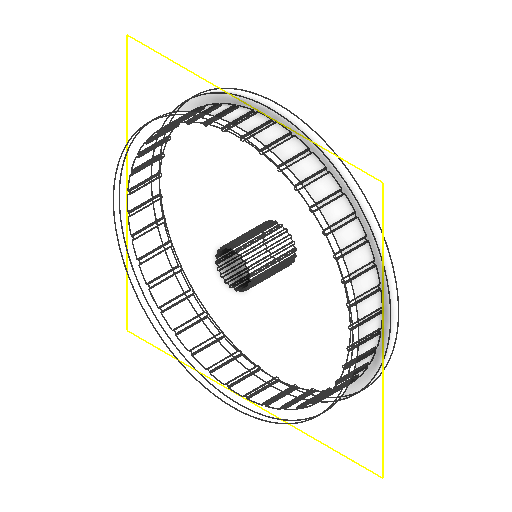
# Autodesk Inventor part: Diff Large Pulley
Saved by Autodesk Inventor 2025.2 (Build 292293000, 293)
## iProperties
Created: 2025-02-20
Part Number: Diff Large Pulley
Material: Generic
Document SubType Name: Modeling
Designer: Jakeg
Density: 1 g/cm^3
Appearance: Default
Author: Jakeg
Autodesk Inventor part; units mm, degrees
ref_plane "YZ Plane" through (0, 0, 0) normal (1, 0, 0) x (0, 1, 0)
ref_plane "XZ Plane" through (0, 0, 0) normal (0, 1, 0) x (-1, 0, 0)
ref_plane "XY Plane" through (0, 0, 0) normal (0, 0, 1) x (1, 0, 0)
sketch "Sketch1" plane through (0, 0, 0) normal (0, 0, 1) x (1, 0, 0)
  circle A0 centre (0, 0) radius 41.14
  dimension "d0" = 82.28
  constraints: 1 centre point, 1 coincident
  measures "d0" diameter of A0
extrude "Extrusion1" add sketch "Sketch1" along normal blind 15.7
ref_plane "Work Plane1" through (0, 0, 8.2) normal (0, 0, 1) x (1, 0, 0)
sketch "Sketch2" plane through (0, 0, 8.2) normal (0, 0, 1) x (1, 0, 0)
  circle A0 centre (0, 0) radius 38.3
  circle A1 centre (0, 0) radius 41.14
  dimension "d4" = 76.6
  constraints: 2 centre point, 2 coincident
  measures "d4" diameter of A0
extrude "Extrusion2" cut sketch "Sketch2" along normal mid plane 11
sketch "Sketch3" plane through (0, 0, 15.7) normal (0, 0, 1) x (1, 0, 0)
  circle A0 centre (0, 0) radius 6
  circle A1 centre (0, 20.32) radius 3.175
  circle A2 centre (0, -20.32) radius 3.175
  dimension "d7" = 12
  dimension "d13" = 6.35
  dimension "d14" = 20.32
  dimension "d15" = 6.35
  dimension "d16" = 20.32
  constraints: 3 centre point, 1 coincident
  measures "d7" diameter of A0
  measures "d13" diameter of A1
  measures "d14" distance of point (0, 0) A1.centre
  measures "d15" diameter of A2
  measures "d16" distance of point (0, 0) A2.centre
extrude "Extrusion3" cut sketch "Sketch3" against normal through all contours A0
sketch "Sketch5" plane through (0, 0, 15.7) normal (0, 0, 1) x (1, 0, 0)
  circle A0 centre (0, 0) radius 6 projected
  arc A1 (-1.2778, -5.5469) -> (-2.2267, -5.2386) centre (-1.8274, -5.6241) ccw
  arc A2 (-1.2783, -5.8289) -> (-1.2778, -5.5469) centre (-2.2681, -5.6859) ccw
  arc A3 (-1.2783, -5.8289) -> (-1.1583, -5.9977) centre (-1.1299, -5.8504) ccw
  arc A4 (-1.1583, -5.9977) -> (-0.7518, -6.0621) centre (0, 0) ccw
  arc A5 (-0.7518, -6.0621) -> (-0.5855, -5.9387) centre (-0.7333, -5.9132) ccw
  arc A6 (-0.4989, -5.6703) -> (-0.5855, -5.9387) centre (0.4, -6.1085) ccw
  arc A7 (0.4989, -5.6703) -> (-0.4989, -5.6703) centre (0, -5.9135) ccw
  arc A8 (0.5855, -5.9387) -> (0.4989, -5.6703) centre (-0.4, -6.1085) ccw
  arc A9 (0.5855, -5.9387) -> (0.7518, -6.0621) centre (0.7333, -5.9132) ccw
  arc A10 (0.7518, -6.0621) -> (1.1583, -5.9977) centre (0, 0) ccw
  arc A11 (1.1583, -5.9977) -> (1.2783, -5.8289) centre (1.1299, -5.8504) ccw
  arc A12 (1.2778, -5.5469) -> (1.2783, -5.8289) centre (2.2681, -5.6859) ccw
  arc A13 (2.2267, -5.2386) -> (1.2778, -5.5469) centre (1.8274, -5.6241) ccw
  arc A14 (2.392, -5.4671) -> (2.2267, -5.2386) centre (1.5072, -5.9331) ccw
  arc A15 (2.392, -5.4671) -> (2.5882, -5.5331) centre (2.5247, -5.3972) ccw
  arc A16 (2.5882, -5.5331) -> (2.955, -5.3462) centre (0, 0) ccw
  arc A17 (2.955, -5.3462) -> (3.017, -5.1486) centre (2.8824, -5.2149) ccw
  arc A18 (2.9293, -4.8806) -> (3.017, -5.1486) centre (3.9141, -4.7068) ccw
  arc A19 (3.7365, -4.2941) -> (2.9293, -4.8806) centre (3.4759, -4.7841) ccw
  arc A20 (3.9643, -4.4604) -> (3.7365, -4.2941) centre (3.2669, -5.177) ccw
  arc A21 (3.9643, -4.4604) -> (4.1714, -4.4624) centre (4.0689, -4.3529) ccw
  arc A22 (4.1714, -4.4624) -> (4.4624, -4.1714) centre (0, 0) ccw
  arc A23 (4.4624, -4.1714) -> (4.4604, -3.9643) centre (4.3529, -4.0689) ccw
  arc A24 (4.2941, -3.7365) -> (4.4604, -3.9643) centre (5.177, -3.2669) ccw
  arc A25 (4.8806, -2.9293) -> (4.2941, -3.7365) centre (4.7841, -3.4759) ccw
  arc A26 (5.1486, -3.017) -> (4.8806, -2.9293) centre (4.7068, -3.9141) ccw
  arc A27 (5.1486, -3.017) -> (5.3462, -2.955) centre (5.2149, -2.8824) ccw
  arc A28 (5.3462, -2.955) -> (5.5331, -2.5882) centre (0, 0) ccw
  arc A29 (5.5331, -2.5882) -> (5.4671, -2.392) centre (5.3972, -2.5247) ccw
  arc A30 (5.2386, -2.2267) -> (5.4671, -2.392) centre (5.9331, -1.5072) ccw
  arc A31 (5.5469, -1.2778) -> (5.2386, -2.2267) centre (5.6241, -1.8274) ccw
  arc A32 (5.8289, -1.2783) -> (5.5469, -1.2778) centre (5.6859, -2.2681) ccw
  arc A33 (5.8289, -1.2783) -> (5.9977, -1.1583) centre (5.8504, -1.1299) ccw
  arc A34 (5.9977, -1.1583) -> (6.0621, -0.7518) centre (0, 0) ccw
  arc A35 (6.0621, -0.7518) -> (5.9387, -0.5855) centre (5.9132, -0.7333) ccw
  arc A36 (5.6703, -0.4989) -> (5.9387, -0.5855) centre (6.1085, 0.4) ccw
  arc A37 (5.6703, 0.4989) -> (5.6703, -0.4989) centre (5.9135, 0) ccw
  arc A38 (5.9387, 0.5855) -> (5.6703, 0.4989) centre (6.1085, -0.4) ccw
  arc A39 (5.9387, 0.5855) -> (6.0621, 0.7518) centre (5.9132, 0.7333) ccw
  arc A40 (6.0621, 0.7518) -> (5.9977, 1.1583) centre (0, 0) ccw
  arc A41 (5.9977, 1.1583) -> (5.8289, 1.2783) centre (5.8504, 1.1299) ccw
  arc A42 (5.5469, 1.2778) -> (5.8289, 1.2783) centre (5.6859, 2.2681) ccw
  arc A43 (5.2386, 2.2267) -> (5.5469, 1.2778) centre (5.6241, 1.8274) ccw
  arc A44 (5.4671, 2.392) -> (5.2386, 2.2267) centre (5.9331, 1.5072) ccw
  arc A45 (5.4671, 2.392) -> (5.5331, 2.5882) centre (5.3972, 2.5247) ccw
  arc A46 (5.5331, 2.5882) -> (5.3462, 2.955) centre (0, 0) ccw
  arc A47 (5.3462, 2.955) -> (5.1486, 3.017) centre (5.2149, 2.8824) ccw
  arc A48 (4.8806, 2.9293) -> (5.1486, 3.017) centre (4.7068, 3.9141) ccw
  arc A49 (4.2941, 3.7365) -> (4.8806, 2.9293) centre (4.7841, 3.4759) ccw
  arc A50 (4.4604, 3.9643) -> (4.2941, 3.7365) centre (5.177, 3.2669) ccw
  arc A51 (4.4604, 3.9643) -> (4.4624, 4.1714) centre (4.3529, 4.0689) ccw
  arc A52 (4.4624, 4.1714) -> (4.1714, 4.4624) centre (0, 0) ccw
  arc A53 (4.1714, 4.4624) -> (3.9643, 4.4604) centre (4.0689, 4.3529) ccw
  arc A54 (3.7365, 4.2941) -> (3.9643, 4.4604) centre (3.2669, 5.177) ccw
  arc A55 (2.9293, 4.8806) -> (3.7365, 4.2941) centre (3.4759, 4.7841) ccw
  arc A56 (3.017, 5.1486) -> (2.9293, 4.8806) centre (3.9141, 4.7068) ccw
  arc A57 (3.017, 5.1486) -> (2.955, 5.3462) centre (2.8824, 5.2149) ccw
  arc A58 (2.955, 5.3462) -> (2.5882, 5.5331) centre (0, 0) ccw
  arc A59 (2.5882, 5.5331) -> (2.392, 5.4671) centre (2.5247, 5.3972) ccw
  arc A60 (2.2267, 5.2386) -> (2.392, 5.4671) centre (1.5072, 5.9331) ccw
  arc A61 (1.2778, 5.5469) -> (2.2267, 5.2386) centre (1.8274, 5.6241) ccw
  arc A62 (1.2783, 5.8289) -> (1.2778, 5.5469) centre (2.2681, 5.6859) ccw
  arc A63 (1.2783, 5.8289) -> (1.1583, 5.9977) centre (1.1299, 5.8504) ccw
  arc A64 (1.1583, 5.9977) -> (0.7518, 6.0621) centre (0, 0) ccw
  arc A65 (0.7518, 6.0621) -> (0.5855, 5.9387) centre (0.7333, 5.9132) ccw
  arc A66 (0.4989, 5.6703) -> (0.5855, 5.9387) centre (-0.4, 6.1085) ccw
  arc A67 (-0.4989, 5.6703) -> (0.4989, 5.6703) centre (0, 5.9135) ccw
  arc A68 (-0.5855, 5.9387) -> (-0.4989, 5.6703) centre (0.4, 6.1085) ccw
  arc A69 (-0.5855, 5.9387) -> (-0.7518, 6.0621) centre (-0.7333, 5.9132) ccw
  arc A70 (-0.7518, 6.0621) -> (-1.1583, 5.9977) centre (0, 0) ccw
  arc A71 (-1.1583, 5.9977) -> (-1.2783, 5.8289) centre (-1.1299, 5.8504) ccw
  arc A72 (-1.2778, 5.5469) -> (-1.2783, 5.8289) centre (-2.2681, 5.6859) ccw
  arc A73 (-2.2267, 5.2386) -> (-1.2778, 5.5469) centre (-1.8274, 5.6241) ccw
  arc A74 (-2.392, 5.4671) -> (-2.2267, 5.2386) centre (-1.5072, 5.9331) ccw
  arc A75 (-2.392, 5.4671) -> (-2.5882, 5.5331) centre (-2.5247, 5.3972) ccw
  arc A76 (-2.5882, 5.5331) -> (-2.955, 5.3462) centre (0, 0) ccw
  arc A77 (-2.955, 5.3462) -> (-3.017, 5.1486) centre (-2.8824, 5.2149) ccw
  arc A78 (-2.9293, 4.8806) -> (-3.017, 5.1486) centre (-3.9141, 4.7068) ccw
  arc A79 (-3.7365, 4.2941) -> (-2.9293, 4.8806) centre (-3.4759, 4.7841) ccw
  arc A80 (-3.9643, 4.4604) -> (-3.7365, 4.2941) centre (-3.2669, 5.177) ccw
  arc A81 (-3.9643, 4.4604) -> (-4.1714, 4.4624) centre (-4.0689, 4.3529) ccw
  arc A82 (-4.1714, 4.4624) -> (-4.4624, 4.1714) centre (0, 0) ccw
  arc A83 (-4.4624, 4.1714) -> (-4.4604, 3.9643) centre (-4.3529, 4.0689) ccw
  arc A84 (-4.2941, 3.7365) -> (-4.4604, 3.9643) centre (-5.177, 3.2669) ccw
  arc A85 (-4.8806, 2.9293) -> (-4.2941, 3.7365) centre (-4.7841, 3.4759) ccw
  arc A86 (-5.1486, 3.017) -> (-4.8806, 2.9293) centre (-4.7068, 3.9141) ccw
  arc A87 (-5.1486, 3.017) -> (-5.3462, 2.955) centre (-5.2149, 2.8824) ccw
  arc A88 (-5.3462, 2.955) -> (-5.5331, 2.5882) centre (0, 0) ccw
  arc A89 (-5.5331, 2.5882) -> (-5.4671, 2.392) centre (-5.3972, 2.5247) ccw
  arc A90 (-5.2386, 2.2267) -> (-5.4671, 2.392) centre (-5.9331, 1.5072) ccw
  arc A91 (-5.5469, 1.2778) -> (-5.2386, 2.2267) centre (-5.6241, 1.8274) ccw
  arc A92 (-5.8289, 1.2783) -> (-5.5469, 1.2778) centre (-5.6859, 2.2681) ccw
  arc A93 (-5.8289, 1.2783) -> (-5.9977, 1.1583) centre (-5.8504, 1.1299) ccw
  arc A94 (-5.9977, 1.1583) -> (-6.0621, 0.7518) centre (0, 0) ccw
  arc A95 (-6.0621, 0.7518) -> (-5.9387, 0.5855) centre (-5.9132, 0.7333) ccw
  arc A96 (-5.6703, 0.4989) -> (-5.9387, 0.5855) centre (-6.1085, -0.4) ccw
  arc A97 (-5.6703, -0.4989) -> (-5.6703, 0.4989) centre (-5.9135, 0) ccw
  arc A98 (-5.9387, -0.5855) -> (-5.6703, -0.4989) centre (-6.1085, 0.4) ccw
  arc A99 (-5.9387, -0.5855) -> (-6.0621, -0.7518) centre (-5.9132, -0.7333) ccw
  arc A100 (-6.0621, -0.7518) -> (-5.9977, -1.1583) centre (0, 0) ccw
  arc A101 (-5.9977, -1.1583) -> (-5.8289, -1.2783) centre (-5.8504, -1.1299) ccw
  arc A102 (-5.5469, -1.2778) -> (-5.8289, -1.2783) centre (-5.6859, -2.2681) ccw
  arc A103 (-5.2386, -2.2267) -> (-5.5469, -1.2778) centre (-5.6241, -1.8274) ccw
  arc A104 (-5.4671, -2.392) -> (-5.2386, -2.2267) centre (-5.9331, -1.5072) ccw
  arc A105 (-5.4671, -2.392) -> (-5.5331, -2.5882) centre (-5.3972, -2.5247) ccw
  arc A106 (-5.5331, -2.5882) -> (-5.3462, -2.955) centre (0, 0) ccw
  arc A107 (-5.3462, -2.955) -> (-5.1486, -3.017) centre (-5.2149, -2.8824) ccw
  arc A108 (-4.8806, -2.9293) -> (-5.1486, -3.017) centre (-4.7068, -3.9141) ccw
  arc A109 (-4.2941, -3.7365) -> (-4.8806, -2.9293) centre (-4.7841, -3.4759) ccw
  arc A110 (-4.4604, -3.9643) -> (-4.2941, -3.7365) centre (-5.177, -3.2669) ccw
  arc A111 (-4.4604, -3.9643) -> (-4.4624, -4.1714) centre (-4.3529, -4.0689) ccw
  arc A112 (-4.4624, -4.1714) -> (-4.1714, -4.4624) centre (0, 0) ccw
  arc A113 (-4.1714, -4.4624) -> (-3.9643, -4.4604) centre (-4.0689, -4.3529) ccw
  arc A114 (-3.7365, -4.2941) -> (-3.9643, -4.4604) centre (-3.2669, -5.177) ccw
  arc A115 (-2.9293, -4.8806) -> (-3.7365, -4.2941) centre (-3.4759, -4.7841) ccw
  arc A116 (-3.017, -5.1486) -> (-2.9293, -4.8806) centre (-3.9141, -4.7068) ccw
  arc A117 (-3.017, -5.1486) -> (-2.955, -5.3462) centre (-2.8824, -5.2149) ccw
  arc A118 (-2.955, -5.3462) -> (-2.5882, -5.5331) centre (0, 0) ccw
  arc A119 (-2.5882, -5.5331) -> (-2.392, -5.4671) centre (-2.5247, -5.3972) ccw
  arc A120 (-2.2267, -5.2386) -> (-2.392, -5.4671) centre (-1.5072, -5.9331) ccw
  point P0 (-3.9904, -4.4807)
  point P1 (-3.0283, -5.1797)
  point P2 (-5.1797, -3.0283)
  point P3 (-4.4807, -3.9904)
  point P4 (-5.862, -1.2794)
  point P5 (-5.4945, -2.4105)
  point P6 (-5.9705, 0.5947)
  point P7 (-5.9705, -0.5947)
  point P8 (-5.4945, 2.4105)
  point P9 (-5.862, 1.2794)
  point P10 (-4.4807, 3.9904)
  point P11 (-5.1797, 3.0283)
  point P12 (-3.0283, 5.1797)
  point P13 (-3.9904, 4.4807)
  point P14 (-1.2794, 5.862)
  point P15 (-2.4105, 5.4945)
  point P16 (0.5947, 5.9705)
  point P17 (-0.5947, 5.9705)
  point P18 (2.4105, 5.4945)
  point P19 (1.2794, 5.862)
  point P20 (3.9904, 4.4807)
  point P21 (3.0283, 5.1797)
  point P22 (5.1797, 3.0283)
  point P23 (4.4807, 3.9904)
  point P24 (5.862, 1.2794)
  point P25 (5.4945, 2.4105)
  point P26 (5.9705, -0.5947)
  point P27 (5.9705, 0.5947)
  point P28 (5.4945, -2.4105)
  point P29 (5.862, -1.2794)
  point P30 (4.4807, -3.9904)
  point P31 (5.1797, -3.0283)
  point P32 (3.0283, -5.1797)
  point P33 (3.9904, -4.4807)
  point P34 (1.2794, -5.862)
  point P35 (2.4105, -5.4945)
  point P36 (-0.5947, -5.9705)
  point P37 (0.5947, -5.9705)
  point P38 (-2.4105, -5.4945)
  point P39 (-1.2794, -5.862)
  dimension "d21" = 0
  dimension "d22" = 0
  constraints: 240 point on circle, 120 centre point, 1 coincident, 1 other
  measures "d21" distance of point (0, 0) A4.centre
  measures "d22" distance of A4.centre point (0, 0)
extrude "Extrusion5" add sketch "Sketch5" against normal blind 15.7 contours A0 A35 A36 A37 A38 A39 | A0 A41 A40 A39 | A35 A34 A33 A0 | A41 A42 A43 A44 A45 A0 | A0 A29 A30 A31 A32 A33 | A0 A47 A46 A45 | A29 A28 A27 A0 | A47 A48 A49 A50 A51 A0 | A0 A23 A24 A25 A26 A27 | A0 A53 A52 A51 | A23 A22 A21 A0 | A53 A54 A55 A56 A57 A0 | A0 A17 A18 A19 A20 A21 | A0 A59 A58 A57 | A17 A16 A15 A0 | A59 A60 A61 A62 A63 A0 | A0 A11 A12 A13 A14 A15 | A0 A65 A64 A63 | A11 A10 A9 A0 | A65 A66 A67 A68 A69 A0 | A0 A5 A6 A7 A8 A9 | A0 A71 A70 A69 | A5 A4 A3 A0 | A71 A72 A73 A74 A75 A0 | A0 A119 A120 A1 A2 A3 | A0 A77 A76 A75 | A119 A118 A117 A0 | A77 A78 A79 A80 A81 A0 | A0 A113 A114 A115 A116 A117 | A0 A83 A82 A81 | A113 A112 A111 A0 | A83 A84 A85 A86 A87 A0 | A0 A107 A108 A109 A110 A111 | A0 A89 A88 A87 | A107 A106 A105 A0 | A89 A90 A91 A92 A93 A0 | A0 A101 A102 A103 A104 A105 | A0 A95 A94 A93 | A101 A100 A99 A0 | A95 A96 A97 A98 A99 A0
sketch "Sketch7" plane through (0, 0, 2.7) normal (0, 0, 1) x (1, 0, 0)
  circle A0 centre (0, 0) radius 38.3
  arc A1 (-34.8303, 15.9293) -> (-34.7968, 15.7578) centre (-34.6939, 15.8669) ccw
  arc A2 (-34.5851, 15.5715) -> (-34.7968, 15.7578) centre (-35.3449, 14.9214) ccw
  arc A3 (-34.9742, 14.6783) -> (-34.5851, 15.5715) centre (-35.0234, 15.2311) ccw
  arc A4 (-35.2563, 14.6789) -> (-34.9742, 14.6783) centre (-35.1132, 15.6686) ccw
  arc A5 (-35.2563, 14.6789) -> (-35.425, 14.5589) centre (-35.2455, 14.4851) ccw
  circle A6 centre (0, 0) radius 38.3 projected
  arc A7 (-37.0213, 9.8138) -> (-36.9594, 9.6505) centre (-36.8763, 9.7754) ccw
  arc A8 (-36.7192, 9.5027) -> (-36.9594, 9.6505) centre (-37.3583, 8.7335) ccw
  arc A9 (-36.9518, 8.5565) -> (-36.7192, 9.5027) centre (-37.0937, 9.093) ccw
  arc A10 (-37.2299, 8.5094) -> (-36.9518, 8.5565) centre (-37.2562, 9.5091) ccw
  arc A11 (-37.2299, 8.5094) -> (-37.3759, 8.3626) centre (-37.1865, 8.3202) ccw
  arc A12 (-38.1474, 3.416) -> (-38.0587, 3.2655) centre (-37.998, 3.4026) ccw
  arc A13 (-37.797, 3.1604) -> (-38.0587, 3.2655) centre (-38.2969, 2.2943) ccw
  arc A14 (-37.8664, 2.1885) -> (-37.797, 3.1604) centre (-38.0969, 2.6934) ccw
  arc A15 (-38.1324, 2.0951) -> (-37.8664, 2.1885) centre (-38.3273, 3.076) ccw
  arc A16 (-38.1324, 2.0951) -> (-38.2516, 1.9258) centre (-38.0577, 1.916) ccw
  arc A17 (-38.176, -3.0801) -> (-38.0631, -3.2134) centre (-38.0264, -3.068) ccw
  arc A18 (-37.7875, -3.2728) -> (-38.0631, -3.2134) centre (-38.1337, -4.2109) ccw
  arc A19 (-37.6915, -4.2424) -> (-37.7875, -3.2728) centre (-38.0041, -3.7838) ccw
  arc A20 (-37.938, -4.3794) -> (-37.6915, -4.2424) centre (-38.2958, -3.4456) ccw
  arc A21 (-37.938, -4.3794) -> (-38.0268, -4.5665) centre (-37.8341, -4.5433) ccw
  arc A22 (-37.1063, -9.4875) -> (-36.9726, -9.5999) centre (-36.961, -9.4504) ccw
  arc A23 (-36.6908, -9.6118) -> (-36.9726, -9.5999) centre (-36.8735, -10.595) ccw
  arc A24 (-36.4324, -10.5513) -> (-36.6908, -9.6118) centre (-36.818, -10.1521) ccw
  arc A25 (-36.6522, -10.728) -> (-36.4324, -10.5513) centre (-37.1627, -9.8681) ccw
  arc A26 (-36.6522, -10.728) -> (-36.7081, -10.9274) centre (-36.522, -10.872) ccw
  arc A27 (-34.9692, -15.622) -> (-34.8184, -15.7102) centre (-34.8322, -15.5609) ccw
  arc A28 (-34.5386, -15.6744) -> (-34.8184, -15.7102) centre (-34.5526, -16.6743) ccw
  arc A29 (-34.1252, -16.5566) -> (-34.5386, -15.6744) centre (-34.5727, -16.2283) ccw
  arc A30 (-34.3119, -16.7679) -> (-34.1252, -16.5566) centre (-34.9604, -16.0067) ccw
  arc A31 (-34.3119, -16.7679) -> (-34.3333, -16.9739) centre (-34.1593, -16.8879) ccw
  arc A32 (-31.826, -21.3071) -> (-31.6625, -21.3686) centre (-31.7014, -21.2237) ccw
  arc A33 (-31.3929, -21.286) -> (-31.6625, -21.3686) centre (-31.2376, -22.2738) ccw
  arc A34 (-30.8363, -22.0856) -> (-31.3929, -21.286) centre (-31.3328, -21.8377) ccw
  arc A35 (-30.9846, -22.3255) -> (-30.8363, -22.0856) centre (-31.7524, -21.6848) ccw
  arc A36 (-30.9846, -22.3255) -> (-30.9709, -22.5321) centre (-30.8139, -22.4179) ccw
  arc A37 (-27.7673, -26.3793) -> (-27.5957, -26.4122) centre (-27.6586, -26.276) ccw
  arc A38 (-27.344, -26.2852) -> (-27.5957, -26.4122) centre (-27.024, -27.2326) ccw
  arc A39 (-26.6602, -26.9793) -> (-27.344, -26.2852) centre (-27.1915, -26.8188) ccw
  arc A40 (-26.7659, -27.2408) -> (-26.6602, -26.9793) centre (-27.6309, -26.739) ccw
  arc A41 (-26.7659, -27.2408) -> (-26.7174, -27.4421) centre (-26.582, -27.303) ccw
  arc A42 (-22.9098, -30.6925) -> (-22.7351, -30.696) centre (-22.8201, -30.5723) ccw
  arc A43 (-22.5084, -30.5283) -> (-22.7351, -30.696) centre (-22.033, -31.408) ccw
  arc A44 (-21.7172, -31.0968) -> (-22.5084, -30.5283) centre (-22.268, -31.0285) ccw
  arc A45 (-21.7772, -31.3724) -> (-21.7172, -31.0968) centre (-22.7146, -31.0241) ccw
  arc A46 (-21.7772, -31.3724) -> (-21.6954, -31.5626) centre (-21.5855, -31.4027) ccw
  arc A47 (-17.3932, -34.1228) -> (-17.2205, -34.0967) centre (-17.3251, -33.9892) ccw
  arc A48 (-17.0254, -33.8931) -> (-17.2205, -34.0967) centre (-16.4081, -34.6798) ccw
  arc A49 (-16.1494, -34.3198) -> (-17.0254, -33.8931) centre (-16.7038, -34.3455) ccw
  arc A50 (-16.162, -34.6015) -> (-16.1494, -34.3198) centre (-17.1447, -34.4166) ccw
  arc A51 (-16.162, -34.6015) -> (-16.0492, -34.7752) centre (-15.9679, -34.5989) ccw
  arc A52 (-11.3762, -36.5715) -> (-11.2104, -36.5165) centre (-11.3316, -36.4282) ccw
  arc A53 (-11.0525, -36.2828) -> (-11.2104, -36.5165) centre (-10.3111, -36.9539) ccw
  arc A54 (-10.1171, -36.5554) -> (-11.0525, -36.2828) centre (-10.6592, -36.6744) ccw
  arc A55 (-10.0818, -36.8352) -> (-10.1171, -36.5554) centre (-11.0817, -36.819) ccw
  arc A56 (-10.0818, -36.8352) -> (-9.9413, -36.9873) centre (-9.891, -36.7998) ccw
  arc A57 (-5.032, -37.968) -> (-4.8778, -37.8858) centre (-5.0123, -37.8193) ccw
  arc A58 (-4.7617, -37.6288) -> (-4.8778, -37.8858) centre (-3.9176, -38.165) ccw
  arc A59 (-3.7937, -37.7394) -> (-4.7617, -37.6288) centre (-4.3078, -37.9483) ccw
  arc A60 (-3.7116, -38.0092) -> (-3.7937, -37.7394) centre (-4.6998, -38.1622) ccw
  arc A61 (-3.7116, -38.0092) -> (-3.5475, -38.1354) centre (-3.5295, -37.9421) ccw
  arc A62 (1.457, -38.2723) -> (1.5951, -38.1652) centre (1.4513, -38.1224) ccw
  arc A63 (1.6661, -37.8923) -> (1.5951, -38.1652) centre (2.5887, -38.2781) ccw
  arc A64 (2.6389, -37.8376) -> (1.6661, -37.8923) centre (2.1674, -38.1304) ccw
  arc A65 (2.7653, -38.0897) -> (2.6389, -37.8376) centre (1.8172, -38.4076) ccw
  arc A66 (2.7653, -38.0897) -> (2.9485, -38.1863) centre (2.9335, -37.9928) ccw
  arc A67 (7.9041, -37.4755) -> (8.0221, -37.3467) centre (7.8732, -37.3288) ccw
  arc A68 (8.046, -37.0657) -> (8.0221, -37.3467) centre (9.0205, -37.29) ccw
  arc A69 (8.9955, -36.8474) -> (8.046, -37.0657) centre (8.5803, -37.2157) ccw
  arc A70 (9.1628, -37.0745) -> (8.9955, -36.8474) centre (8.282, -37.548) ccw
  arc A71 (9.1628, -37.0745) -> (9.3596, -37.1388) centre (9.3122, -36.9506) ccw
  arc A72 (14.1238, -35.6007) -> (14.2183, -35.4537) centre (14.0685, -35.4612) ccw
  arc A73 (14.1944, -35.1728) -> (14.2183, -35.4537) centre (15.1928, -35.2291) ccw
  arc A74 (15.0934, -34.7971) -> (14.1944, -35.1728) centre (14.7464, -35.2303) ccw
  arc A75 (15.2966, -34.9927) -> (15.0934, -34.7971) centre (14.5085, -35.6083) ccw
  arc A76 (15.2966, -34.9927) -> (15.5014, -35.0228) centre (15.4229, -34.8453) ccw
  arc A77 (19.9372, -32.7016) -> (20.0055, -32.5409) centre (19.8591, -32.5736) ccw
  arc A78 (19.9344, -32.268) -> (20.0055, -32.5409) centre (20.928, -32.1548) ccw
  arc A79 (20.757, -31.7458) -> (19.9344, -32.268) centre (20.4882, -32.2314) ccw
  arc A80 (20.9903, -31.9042) -> (20.757, -31.7458) centre (20.3176, -32.6441) ccw
  arc A81 (20.9903, -31.9042) -> (21.1973, -31.8993) centre (21.0899, -31.7376) ccw
  arc A82 (25.177, -28.8619) -> (25.2172, -28.6918) centre (25.0784, -28.7488) ccw
  arc A83 (25.101, -28.4349) -> (25.2172, -28.6918) centre (26.0612, -28.1554) ccw
  arc A84 (25.8235, -27.7812) -> (25.101, -28.4349) centre (25.6406, -28.3052) ccw
  arc A85 (26.0803, -27.8979) -> (25.8235, -27.7812) centre (25.5423, -28.7409) ccw
  arc A86 (26.0803, -27.8979) -> (26.2834, -27.858) centre (26.1502, -27.7169) ccw
  arc A87 (29.6926, -24.1918) -> (29.7034, -24.0174) centre (29.5763, -24.097) ccw
  arc A88 (29.5455, -23.7838) -> (29.7034, -24.0174) centre (30.4446, -23.3461) ccw
  arc A89 (30.1471, -23.0174) -> (29.5455, -23.7838) centre (30.0554, -23.5648) ccw
  arc A90 (30.4199, -23.089) -> (30.1471, -23.0174) centre (30.0321, -24.0108) ccw
  arc A91 (30.4199, -23.089) -> (30.6134, -23.0154) centre (30.4583, -22.8988) ccw
  arc A92 (33.3539, -18.8257) -> (33.3351, -18.652) centre (33.2233, -18.752) ccw
  arc A93 (33.14, -18.4485) -> (33.3351, -18.652) centre (33.9522, -17.8651) ccw
  arc A94 (33.6034, -17.5914) -> (33.14, -18.4485) centre (33.6056, -18.1464) ccw
  arc A95 (33.8844, -17.6159) -> (33.6034, -17.5914) centre (33.6579, -18.59) ccw
  arc A96 (33.8844, -17.6159) -> (34.0627, -17.5107) centre (33.8901, -17.4219) ccw
  arc A97 (36.0557, -12.9181) -> (36.0078, -12.7501) centre (35.9145, -12.8675) ccw
  arc A98 (35.7811, -12.5824) -> (36.0078, -12.7501) centre (36.483, -11.8702) ccw
  arc A99 (36.0931, -11.6594) -> (35.7811, -12.5824) centre (36.189, -12.2061) ccw
  arc A100 (36.3741, -11.6361) -> (36.0931, -11.6594) centre (36.3155, -12.6343) ccw
  arc A101 (36.3741, -11.6361) -> (36.532, -11.5022) centre (36.3469, -11.4439) ccw
  arc A102 (37.7202, -6.6388) -> (37.6447, -6.4813) centre (37.5725, -6.6128) ccw
  arc A103 (37.3928, -6.3544) -> (37.6447, -6.4813) centre (37.9643, -5.5338) ccw
  arc A104 (37.5443, -5.3919) -> (37.3928, -6.3544) centre (37.7312, -5.9145) ccw
  arc A105 (37.8174, -5.3214) -> (37.5443, -5.3919) centre (37.9284, -6.3153) ccw
  arc A106 (37.8174, -5.3214) -> (37.9504, -5.1628) centre (37.7581, -5.1366) ccw
  arc A107 (38.2996, -0.1686) -> (38.1985, -0.0261) centre (38.1496, -0.1679) ccw
  arc A108 (37.9289, 0.0564) -> (38.1985, -0.0261) centre (38.3535, 0.9618) ccw
  arc A109 (37.9155, 1.0306) -> (37.9289, 0.0564) centre (38.1881, 0.5472) ccw
  arc A110 (38.1728, 1.1463) -> (37.9155, 1.0306) centre (38.4501, 0.1855) ccw
  arc A111 (38.1728, 1.1463) -> (38.2771, 1.3251) centre (38.0831, 1.3184) ccw
  arc A112 (37.7772, 6.3065) -> (37.6535, 6.4298) centre (37.6293, 6.2818) ccw
  arc A113 (37.3738, 6.4656) -> (37.6535, 6.4298) centre (37.6392, 7.4297) ccw
  arc A114 (37.196, 7.4236) -> (37.3738, 6.4656) centre (37.5463, 6.9931) ccw
  arc A115 (37.4299, 7.581) -> (37.196, 7.4236) centre (37.8657, 6.6809) ccw
  arc A116 (37.4299, 7.581) -> (37.5025, 7.7749) centre (37.3125, 7.7355) ccw
  arc A117 (36.168, 12.6002) -> (36.0252, 12.7008) centre (36.0264, 12.5508) ccw
  arc A118 (35.7435, 12.6888) -> (36.0252, 12.7008) centre (35.8422, 13.6839) ccw
  arc A119 (35.4064, 13.6029) -> (35.7435, 12.6888) centre (35.8244, 13.2379) ccw
  arc A120 (35.6104, 13.7977) -> (35.4064, 13.6029) centre (36.1919, 12.9842) ccw
  arc A121 (35.6104, 13.7977) -> (35.6491, 14.0011) centre (35.4685, 13.9301) ccw
  arc A122 (33.5183, 18.5314) -> (33.3606, 18.6064) centre (33.3871, 18.4588) ccw
  arc A123 (33.0849, 18.547) -> (33.3606, 18.6064) centre (33.014, 19.5445) ccw
  arc A124 (32.5982, 19.391) -> (33.0849, 18.547) centre (33.0719, 19.1018) ccw
  arc A125 (32.7663, 19.6174) -> (32.5982, 19.391) centre (33.477, 18.9139) ccw
  arc A126 (32.7663, 19.6174) -> (32.7702, 19.8244) centre (32.6041, 19.7239) ccw
  arc A127 (29.9044, 23.9294) -> (29.7362, 23.9768) centre (29.7873, 23.8357) ccw
  arc A128 (29.4746, 23.8716) -> (29.7362, 23.9768) centre (29.2361, 24.8427) ccw
  arc A129 (28.8522, 24.6212) -> (29.4746, 23.8716) centre (29.3679, 24.4162) ccw
  arc A130 (28.9796, 24.8727) -> (28.8522, 24.6212) centre (29.799, 24.2995) ccw
  arc A131 (28.9796, 24.8727) -> (28.9484, 25.0774) centre (28.8017, 24.9503) ccw
  arc A132 (25.4302, 28.6391) -> (25.2564, 28.6573) centre (25.3306, 28.5269) ccw
  arc A133 (25.0163, 28.5094) -> (25.2564, 28.6573) centre (24.6172, 29.4263) ccw
  arc A134 (24.2762, 29.1431) -> (25.0163, 28.5094) centre (24.8192, 29.0282) ccw
  arc A135 (24.3593, 29.4125) -> (24.2762, 29.1431) centre (25.2637, 28.986) ccw
  arc A136 (24.3593, 29.4125) -> (24.2939, 29.609) centre (24.1708, 29.459) ccw
  arc A137 (20.2243, 32.5249) -> (20.05, 32.5135) centre (20.1451, 32.3975) ccw
  arc A138 (19.8384, 32.3271) -> (20.05, 32.5135) centre (19.29, 33.1634) ccw
  arc A139 (19.0018, 32.8266) -> (19.8384, 32.3271) centre (19.5564, 32.8051) ccw
  arc A140 (19.0382, 33.1062) -> (19.0018, 32.8266) centre (20.0017, 32.8386) ccw
  arc A141 (19.0382, 33.1062) -> (18.9405, 33.2888) centre (18.8446, 33.1201) ccw
  arc A142 (14.4367, 35.4749) -> (14.2668, 35.4343) centre (14.3802, 35.336) ccw
  arc A143 (14.0897, 35.2148) -> (14.2668, 35.4343) centre (13.4079, 35.9464) ccw
  arc A144 (13.1807, 35.5657) -> (14.0897, 35.2148) centre (13.731, 35.6383) ccw
  arc A145 (13.1693, 35.8475) -> (13.1807, 35.5657) centre (14.1642, 35.7466) ccw
  arc A146 (13.1693, 35.8475) -> (13.0423, 36.011) centre (12.9762, 35.8285) ccw
  arc A147 (8.2337, 37.4045) -> (8.0732, 37.3357) centre (8.2015, 37.258) ccw
  arc A148 (7.9357, 37.0895) -> (8.0732, 37.3357) centre (7.1401, 37.6953) ccw
  arc A149 (6.9805, 37.2817) -> (7.9357, 37.0895) centre (7.5105, 37.4462) ccw
  arc A150 (6.9217, 37.5575) -> (6.9805, 37.2817) centre (7.9193, 37.6262) ccw
  arc A151 (6.9217, 37.5575) -> (6.7688, 37.6971) centre (6.7345, 37.5061) ccw
  arc A152 (1.7939, 38.258) -> (1.6473, 38.163) centre (1.7869, 38.1081) ccw
  arc A153 (1.5534, 37.8971) -> (1.6473, 38.163) centre (0.6668, 38.3597) ccw
  arc A154 (0.5795, 37.9251) -> (1.5534, 37.8971) centre (1.0741, 38.1769) ccw
  arc A155 (0.4748, 38.187) -> (0.5795, 37.9251) centre (1.4465, 38.4233) ccw
  arc A156 (0.4748, 38.187) -> (0.3006, 38.2988) centre (0.2991, 38.1047) ccw
  arc A157 (-4.6975, 38.0108) -> (-4.826, 37.8925) centre (-4.6791, 37.862) ccw
  arc A158 (-4.8736, 37.6145) -> (-4.826, 37.8925) centre (-5.8256, 37.9206) ccw
  arc A159 (-5.8382, 37.4775) -> (-4.8736, 37.6145) centre (-5.3933, 37.8093) ccw
  arc A160 (-5.9856, 37.718) -> (-5.8382, 37.4775) centre (-5.0679, 38.1151) ccw
  arc A161 (-5.9856, 37.718) -> (-6.1763, 37.7987) centre (-6.145, 37.6072) ccw
  arc A162 (-11.0538, 36.6702) -> (-11.1604, 36.5318) centre (-11.0105, 36.5266) ccw
  arc A163 (-11.1604, 36.2498) -> (-11.1604, 36.5318) centre (-12.1504, 36.3907) ccw
  arc A164 (-12.088, 35.9518) -> (-11.1604, 36.2498) centre (-11.7055, 36.3539) ccw
  arc A165 (-12.2739, 36.1639) -> (-12.088, 35.9518) centre (-11.4364, 36.7104) ccw
  arc A166 (-12.2739, 36.1639) -> (-12.4755, 36.2112) centre (-12.4122, 36.0277) ccw
  arc A167 (-17.0921, 34.2746) -> (-17.1738, 34.1202) centre (-17.0252, 34.1404) ccw
  arc A168 (-17.1261, 33.8423) -> (-17.1738, 34.1202) centre (-18.1257, 33.8138) ccw
  arc A169 (-17.99, 33.3918) -> (-17.1261, 33.8423) centre (-17.681, 33.8528) ccw
  arc A170 (-18.2091, 33.5694) -> (-17.99, 33.3918) centre (-17.476, 34.2496) ccw
  arc A171 (-18.2091, 33.5694) -> (-18.4157, 33.582) centre (-18.3224, 33.4118) ccw
  arc A172 (-22.6387, 30.893) -> (-22.6931, 30.727) centre (-22.55, 30.772) ccw
  arc A173 (-22.5991, 30.4612) -> (-22.6931, 30.727) centre (-23.5795, 30.2641) ccw
  arc A174 (-23.3745, 29.8711) -> (-22.5991, 30.4612) centre (-23.1478, 30.3777) ccw
  arc A175 (-23.6204, 30.0092) -> (-23.3745, 29.8711) centre (-23.0129, 30.8035) ccw
  arc A176 (-23.6204, 30.0092) -> (-23.8262, 29.9867) centre (-23.7055, 29.8347) ccw
  arc A177 (-27.534, 26.6227) -> (-27.5596, 26.4499) centre (-27.4262, 26.5184) ccw
  arc A178 (-27.422, 26.2037) -> (-27.5596, 26.4499) centre (-28.355, 25.8439) ccw
  arc A179 (-28.0865, 25.4912) -> (-27.422, 26.2037) centre (-27.9487, 26.0288) ccw
  arc A180 (-28.3522, 25.5856) -> (-28.0865, 25.4912) centre (-27.8876, 26.4712) ccw
  arc A181 (-28.3522, 25.5856) -> (-28.5513, 25.5287) centre (-28.4066, 25.3993) ccw
  arc A182 (-31.6372, 21.5865) -> (-31.6332, 21.4119) centre (-31.5133, 21.502) ccw
  arc A183 (-31.456, 21.1925) -> (-31.6332, 21.4119) centre (-32.3148, 20.6801) ccw
  arc A184 (-31.9905, 20.3778) -> (-31.456, 21.1925) centre (-31.9456, 20.931) ccw
  arc A185 (-32.2684, 20.4261) -> (-31.9905, 20.3778) centre (-31.9602, 21.3774) ccw
  arc A186 (-32.2684, 20.4261) -> (-32.455, 20.3363) centre (-32.2905, 20.2332) ccw
  point P0 (0, 0)
  point P1 (-31.6372, 21.5865)
  point P2 (-32.455, 20.3363)
  point P3 (-27.534, 26.6227)
  point P4 (-28.5513, 25.5287)
  point P5 (-22.6387, 30.893)
  point P6 (-23.8262, 29.9867)
  point P7 (-17.0921, 34.2746)
  point P8 (-18.4157, 33.582)
  point P9 (-11.0538, 36.6702)
  point P10 (-12.4755, 36.2112)
  point P11 (-4.6975, 38.0108)
  point P12 (-6.1763, 37.7987)
  point P13 (-5.032, -37.968)
  point P14 (-3.5475, -38.1354)
  point P15 (-9.9413, -36.9873)
  point P16 (-17.3932, -34.1228)
  point P17 (-16.0492, -34.7752)
  point P18 (-22.9098, -30.6925)
  point P19 (-21.6954, -31.5626)
  point P20 (-27.7673, -26.3793)
  point P21 (-26.7174, -27.4421)
  point P22 (-31.826, -21.3071)
  point P23 (-30.9709, -22.5321)
  point P24 (-34.9692, -15.622)
  point P25 (-34.3333, -16.9739)
  point P26 (-37.1063, -9.4875)
  point P27 (-36.7081, -10.9274)
  point P28 (-38.176, -3.0801)
  point P29 (-38.0268, -4.5665)
  point P30 (-38.1474, 3.416)
  point P31 (-38.2516, 1.9258)
  point P32 (-37.0213, 9.8138)
  point P33 (-37.3759, 8.3626)
  point P34 (-34.8303, 15.9293)
  point P35 (-35.425, 14.5589)
  point P36 (1.7939, 38.258)
  point P37 (0.3006, 38.2988)
  point P38 (8.2337, 37.4045)
  point P39 (6.7688, 37.6971)
  point P40 (14.4367, 35.4749)
  point P41 (13.0423, 36.011)
  point P42 (20.2243, 32.5249)
  point P43 (18.9405, 33.2888)
  point P44 (25.4302, 28.6391)
  point P45 (24.2939, 29.609)
  point P46 (29.9044, 23.9294)
  point P47 (28.9484, 25.0774)
  point P48 (32.7702, 19.8244)
  point P49 (36.168, 12.6002)
  point P50 (35.6491, 14.0011)
  point P51 (37.7772, 6.3065)
  point P52 (37.5025, 7.7749)
  point P53 (38.2996, -0.1686)
  point P54 (38.2771, 1.3251)
  point P55 (37.7202, -6.6388)
  point P56 (37.9504, -5.1628)
  point P57 (36.0557, -12.9181)
  point P58 (36.532, -11.5022)
  point P59 (33.3539, -18.8257)
  point P60 (34.0627, -17.5107)
  point P61 (29.6926, -24.1918)
  point P62 (30.6134, -23.0154)
  point P63 (25.177, -28.8619)
  point P64 (26.2834, -27.858)
  point P65 (19.9372, -32.7016)
  point P66 (21.1973, -31.8993)
  point P67 (15.5014, -35.0228)
  point P68 (7.9041, -37.4755)
  point P69 (9.3596, -37.1388)
  point P70 (1.457, -38.2723)
  point P71 (2.9485, -38.1863)
  dimension "d30" = 76.6
  dimension "d35" = 360
  constraints: 370 point on circle, 185 centre point, 2 tangent, 594 other
extrude "Extrusion6" cut sketch "Sketch7" along normal blind 11 contours A0 A107 A108 A109 A110 A111 | A112 A113 A114 A115 A116 A0 | A0 A102 A103 A104 A105 A106 | A117 A118 A119 A120 A121 A0 | A0 A97 A98 A99 A100 A101 | A122 A123 A124 A125 A126 A0 | A0 A92 A93 A94 A95 A96 | A127 A128 A129 A130 A131 A0 | A0 A87 A88 A89 A90 A91 | A132 A133 A134 A135 A136 A0 | A0 A82 A83 A84 A85 A86 | A137 A138 A139 A140 A141 A0 | A0 A77 A78 A79 A80 A81 | A142 A143 A144 A145 A146 A0 | A0 A72 A73 A74 A75 A76 | A147 A148 A149 A150 A151 A0 | A0 A67 A68 A69 A70 A71 | A152 A153 A154 A155 A156 A0 | A0 A62 A63 A64 A65 A66 | A157 A158 A159 A160 A161 A0 | A0 A57 A58 A59 A60 A61 | A162 A163 A164 A165 A166 A0 | A0 A52 A53 A54 A55 A56 | A167 A168 A169 A170 A171 A0 | A0 A47 A48 A49 A50 A51 | A172 A173 A174 A175 A176 A0 | A0 A42 A43 A44 A45 A46 | A177 A178 A179 A180 A181 A0 | A0 A37 A38 A39 A40 A41 | A182 A183 A184 A185 A186 A0 | A0 A32 A33 A34 A35 A36 | A1 A2 A3 A4 A5 A0 | A0 A27 A28 A29 A30 A31 | A7 A8 A9 A10 A11 A0 | A0 A22 A23 A24 A25 A26 | A12 A13 A14 A15 A16 A0 | A0 A17 A18 A19 A20 A21
body "Solid1"
